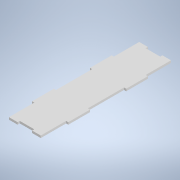
# Autodesk Inventor part: LongSide
Saved by Autodesk Inventor 2020.3 (Build 243373000, 373)
## iProperties
Created: 2020-08-22
Part Number: LongSide
Material: Generic
Document SubType Name: Modeling
Designer: Scott Hanson
Density: 1 g/cm^3
Appearance: Default
Author: Scott Hanson
Autodesk Inventor part; units mm, degrees
ref_plane "YZ Plane" through (0, 0, 0) normal (1, 0, 0) x (0, 1, 0)
ref_plane "XZ Plane" through (0, 0, 0) normal (0, 1, 0) x (-1, 0, 0)
ref_plane "XY Plane" through (0, 0, 0) normal (0, 0, 1) x (1, 0, 0)
sketch "Sketch1" plane through (0, 0, 0) normal (0, 1, 0) x (-1, 0, 0)
  line L0 (0, 0) -> (-50, 0)
  line L1 (-50, 0) -> (-50, -180)
  line L2 (-50, -180) -> (0, -180)
  line L3 (0, -180) -> (0, 0)
  dimension "d0" = 180
  dimension "d1" = 50
  constraints: 8 end point, 2 parallel, 1 horizontal, 1 perpendicular
  measures "d0" distance of L2.end L0.start
  measures "d1" distance of L0.start L0.end
extrude "Base" add sketch "Sketch1" along normal blind 3
sketch "Sketch2" plane through (0, 3, 0) normal (0, 1, 0) x (1, 0, 0)
  line L0 (0, 0) -> (50, 0) projected
  line L1 (50, 180) -> (0, 180) projected
  line L2 (0, 0) -> (3, 0)
  line L3 (3, 180) -> (0, 180)
  line L4 (0, 180) -> (0, 0)
  line L5 (0, 180) -> (0, 0) projected
  line L6 (0, 0) -> (3, 0)
  line L7 (3, 0) -> (3, 35)
  line L8 (3, 35) -> (0, 35)
  line L9 (0, 35) -> (0, 0)
  line L10 (0, 180) -> (3, 180)
  line L11 (3, 180) -> (3, 145)
  line L12 (3, 145) -> (0, 145)
  line L13 (0, 145) -> (0, 180)
  line L14 (0, 65) -> (3, 65)
  line L15 (3, 65) -> (3, 115)
  line L16 (3, 115) -> (0, 115)
  line L17 (0, 115) -> (0, 65)
  line L18 (25, 0) -> (25, 180) construction
  line L19 (50, 0) -> (47, 0)
  line L20 (47, 180) -> (50, 180)
  line L21 (50, 180) -> (50, 0)
  line L22 (50, 180) -> (50, 0)
  line L23 (50, 0) -> (47, 0)
  line L24 (47, 0) -> (47, 35)
  line L25 (47, 35) -> (50, 35)
  line L26 (50, 35) -> (50, 0)
  line L27 (50, 180) -> (47, 180)
  line L28 (47, 180) -> (47, 145)
  line L29 (47, 145) -> (50, 145)
  line L30 (50, 145) -> (50, 180)
  line L31 (50, 65) -> (47, 65)
  line L32 (47, 65) -> (47, 115)
  line L33 (47, 115) -> (50, 115)
  line L34 (50, 115) -> (50, 65)
  line L35 (15, 0) -> (35, 0)
  line L36 (35, 0) -> (35, 3)
  line L37 (35, 3) -> (15, 3)
  line L38 (15, 3) -> (15, 0)
  line L39 (0, 90) -> (50, 90) construction
  line L40 (50, 0) -> (50, 180) projected
  line L41 (35, 180) -> (35, 177)
  line L42 (35, 177) -> (15, 177)
  line L43 (15, 177) -> (15, 180)
  point P0 (0, 145)
  point P1 (0, 115)
  dimension "d10" = 35
  dimension "d11" = 35
  dimension "d12" = 30
  dimension "d13" = 30
  dimension "d14" = 50
  dimension "d15" = 3
  dimension "d18" = 20
  dimension "d19" = 10
  dimension "d20" = 3
  constraints: 80 end point, 18 symmetric about line, 9 parallel, 8 point on line, 5 horizontal, 4 perpendicular, 3 midpoint, 2 other
  measures "d10" distance of L6.end L7.end
  measures "d11" distance of L10.end L11.end
  measures "d12" distance between parallel lines of L14 L8
  measures "d13" distance between parallel lines of L16 L12
  measures "d14" distance of L14.end L15.end
  measures "d15" distance of L7.end L8.end
  measures "d18" distance of L36.end L37.end
  measures "d19" distance from line of L18 L37.end
  measures "d20" distance of L35.end L36.end
extrude "Tabs" cut sketch "Sketch2" against normal through all contours L4 L8 L7 L0 | L38 L37 L36 L0 | L4 L16 L15 L14 | L24 L25 L21 L0 | L4 L1 L11 L12 | L31 L32 L33 L21 | L1 L41 L42 L43 | L29 L28 L1 L21
equation "\"d11\" = d10"
equation "\"d13\" = d12"
equation "\"d19\" = 0.5 * d18"
equation "\"d20\" = d15"
body "Solid1"
